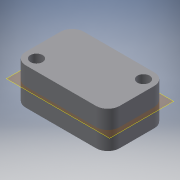
# Autodesk Inventor part: LimitSwitch
Saved by Autodesk Inventor 2019 (Build 230136000, 136)
## iProperties
Created: 2019-01-18
Part Number: LimitSwitch
Material: Generic
Document SubType Name: Modeling
Designer: nxgam
Density: 1 g/cm^3
Appearance: Default
Author: nxgam
Autodesk Inventor part; units mm, degrees
ref_plane "YZ Plane" through (0, 0, 0) normal (1, 0, 0) x (0, 1, 0)
ref_plane "XZ Plane" through (0, 0, 0) normal (0, 1, 0) x (-1, 0, 0)
ref_plane "XY Plane" through (0, 0, 0) normal (0, 0, 1) x (1, 0, 0)
sketch "Sketch1" plane through (0, 0, 0) normal (0, 1, 0) x (-1, 0, 0)
  line L0 (0, 0) -> (25.4, 0)
  line L1 (25.4, 0) -> (25.4, -15.748)
  line L2 (25.4, -15.748) -> (0, -15.748)
  line L3 (0, -15.748) -> (0, 0)
  dimension "d0" = 25.4
  dimension "d1" = 15.748
  constraints: 8 end point, 2 parallel, 1 horizontal, 1 perpendicular
  measures "d0" distance of L1.end L2.end
  measures "d1" distance of L0.end L1.end
extrude "Extrusion1" add sketch "Sketch1" along normal blind 9.906
sketch "Sketch2" plane through (0, 9.906, 0) normal (0, 1, 0) x (1, 0, 0)
  line L0 (-25.4, 0) -> (0, 0) projected
  line L1 (0, 0) -> (0, 15.748) projected
  line L2 (0, 15.748) -> (-25.4, 15.748) projected
  line L3 (-25.4, 15.748) -> (-25.4, 0) projected
  point P0 (-3.048, 12.7)
  point P1 (-22.352, 3.048)
  dimension "d5" = 3.048
  dimension "d6" = 3.048
  dimension "d7" = 3.048
  dimension "d8" = 3.048
  measures "d5" distance from line of L3 point (-22.352, 3.048)
  measures "d6" distance from line of L0 point (-22.352, 3.048)
  measures "d7" distance from line of point (-3.048, 12.7) L2
  measures "d8" distance from line of point (-3.048, 12.7) L1
hole "Hole1" at (-3.048, 9.906, -12.7) at (-22.352, 9.906, -3.048) direction (0, -1, 0) diameter 3.302 end through all
fillet "Fillet1" radius 3.175 4 edges at (-25.4, 4.953, 0) (-25.4, 4.953, -15.748) (0, 4.953, -15.748) (0, 4.953, 0)
ref_plane "Work Plane1" through (0, 4.953, 0) normal (0, 1, 0) x (1, 0, 0)
equation "\"d6\" = d5"
equation "\"d7\" = d6"
equation "\"d8\" = d7"
body "Solid1"
